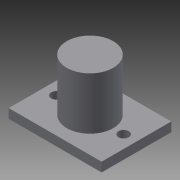
# Autodesk Inventor part: half_inch_castor
Saved by Autodesk Inventor 2015 (Build 190159000, 159)
## iProperties
Created: 2014-11-12
Part Number: half_inch_castor
Material: Generic
Document SubType Name: Modeling
Designer: Colin
Density: 1 g/cm^3
Appearance: Default
Author: Colin
Autodesk Inventor part; units mm, degrees
ref_plane "YZ Plane" through (0, 0, 0) normal (1, 0, 0) x (0, 1, 0)
ref_plane "XZ Plane" through (0, 0, 0) normal (0, 1, 0) x (-1, 0, 0)
ref_plane "XY Plane" through (0, 0, 0) normal (0, 0, 1) x (1, 0, 0)
sketch "Sketch1" plane through (0, 0, 0) normal (0, 1, 0) x (-1, 0, 0)
  line L0 (0, 0) -> (-20.32, 0)
  line L1 (-20.32, 0) -> (-20.32, -15.24)
  line L2 (-20.32, -15.24) -> (0, -15.24)
  line L3 (0, -15.24) -> (0, 0)
  line L4 (-20.32, -7.62) -> (0, -7.62) construction
  circle A0 centre (-17.526, -7.62) radius 1.143
  circle A1 centre (-2.794, -7.62) radius 1.143
  dimension "d0" = 20.32
  dimension "d1" = 15.24
  dimension "d2" = 14.732
  dimension "d3" = 2.794
  dimension "d4" = 2.286
  dimension "d5" = 2.286
  constraints: 10 end point, 2 centre point, 2 midpoint, 2 parallel, 2 point on line, 1 horizontal, 1 perpendicular
  measures "d0" distance of L0.start L0.end
  measures "d1" distance of L0.end L1.end
  measures "d2" distance of A0.centre A1.centre
  measures "d3" distance from line of L3 A1.centre
  measures "d4" diameter of A1
  measures "d5" diameter of A0
extrude "Extrusion1" add sketch "Sketch1" along normal blind 2.032
sketch "Sketch2" plane through (0, 2.032, 0) normal (0, 1, 0) x (1, 0, 0)
  line L0 (0, 15.24) -> (0, 0) construction
  line L1 (0, 7.62) -> (20.32, 7.62) construction
  line L2 (20.32, 0) -> (20.32, 15.24) construction
  line L3 (20.32, 15.24) -> (0, 15.24) construction
  line L4 (10.16, 15.24) -> (10.16, 0) construction
  line L5 (0, 0) -> (20.32, 0) construction
  circle A0 centre (10.16, 7.62) radius 5.08
  dimension "d8" = 10.16
  constraints: 5 midpoint, 4 end point, 1 centre point
  measures "d8" diameter of A0
extrude "Extrusion2" add sketch "Sketch2" along normal blind 11.43
body "Solid1"
